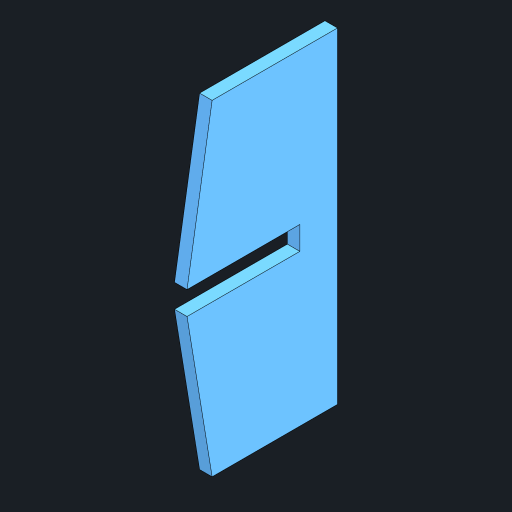
# Autodesk Inventor part: VertWing
Saved by Autodesk Inventor 2023 (Build 270158000, 158)
## iProperties
Created: 2022-06-06
Part Number: VertWing
Material: スタイロフォームIB
Document SubType Name: Modeling
Designer: neko2
Density: 0.027 g/cm^3
Appearance: スタイロフォームIB
Mass: 0.631058 g
Surface Area: 112.411 cm^2
Volume: 23.3725 cm^3
Author: neko2
Autodesk Inventor part; units mm, degrees
ref_plane "YZ Plane" through (0, 0, 0) normal (1, 0, 0) x (0, 1, 0)
ref_plane "XZ Plane" through (0, 0, 0) normal (0, 1, 0) x (-1, 0, 0)
ref_plane "XY Plane" through (0, 0, 0) normal (0, 0, 1) x (1, 0, 0)
sketch "スケッチ1" plane through (0, 0, 0) normal (1, 0, 0) x (0, 1, 0)
  line L0 (0, 0) -> (0, -113.3816)
  line L1 (4.65, 0) -> (65, -10)
  line L2 (65, -10) -> (65, -60)
  line L3 (65, -60) -> (0, -60)
  line L4 (0, 0) -> (0, -30)
  line L5 (0, -60) -> (0, -70)
  line L6 (4.65, 0) -> (4.65, -45)
  line L7 (4.65, -45) -> (0, -45)
  line L8 (-4.65, 0) -> (-65, -10)
  line L9 (-65, -10) -> (-65, -60)
  line L10 (-65, -60) -> (0, -60)
  line L11 (-4.65, 0) -> (-4.65, -45)
  line L12 (-4.65, -45) -> (0, -45)
  dimension "d0" = 4.65
  dimension "d1" = 130
  dimension "d2" = 60
  dimension "d6" = 45
  dimension "d12" = 10
  constraints: 26 end point, 4 point on line, 4 symmetric about line, 3 vertical, 2 perpendicular, 1 horizontal alignment
  measures "d0" horizontal distance of L3.end L1.start
  measures "d1" diameter of L2.end L0
  measures "d2" vertical distance of L0.start L2.end
  measures "d6" distance of L1.start L6.end
  measures "d12" vertical distance of L0.start L1.end
extrude "押し出し1" add sketch "スケッチ1" along normal blind 5
